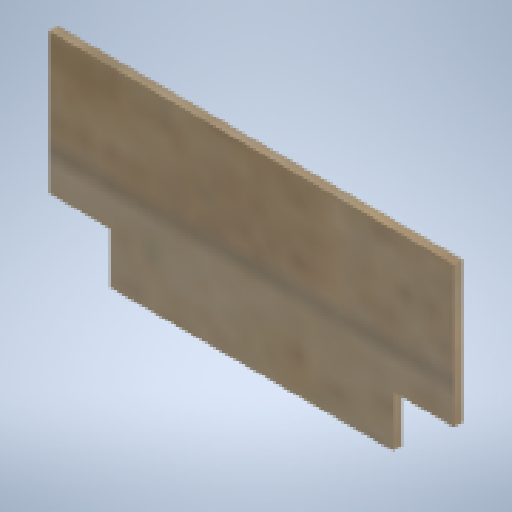
# Autodesk Inventor part: wall
Saved by Autodesk Inventor 2026.1 (Build 301233020, 233B)
## iProperties
Created: 2025-11-03
Part Number: wall
Material: 木材 (カエデ材)
Document SubType Name: Modeling
Designer: hibik
Density: 0.67 g/cm^3
Appearance: ナチュラル カエデ材 - 光沢 濃い着色
Author: hibik
Autodesk Inventor part; units mm, degrees
ref_plane "YZ Plane" through (0, 0, 0) normal (1, 0, 0) x (0, 1, 0)
ref_plane "XZ Plane" through (0, 0, 0) normal (0, 1, 0) x (-1, 0, 0)
ref_plane "XY Plane" through (0, 0, 0) normal (0, 0, 1) x (1, 0, 0)
sketch "スケッチ1" plane through (0, 0, 0) normal (0, 0, 1) x (1, 0, 0)
  line L0 (-40.22, 0) -> (40.22, 0)
  line L1 (40.22, 0) -> (40.22, 14.5)
  line L2 (40.22, 14.5) -> (-40.22, 14.5)
  line L3 (-40.22, 14.5) -> (-40.22, 0)
  line L4 (-57.5, 14.5) -> (57.5, 14.5)
  line L5 (57.5, 14.5) -> (57.5, 54.5)
  line L6 (57.5, 54.5) -> (-57.5, 54.5)
  line L7 (-57.5, 54.5) -> (-57.5, 14.5)
  point P0 (0, 0)
  point P1 (0, 0)
  point P2 (0, 14.5)
  dimension "d0" = 80.44
  dimension "d1" = 14.5
  dimension "d2" = 115
  dimension "d3" = 40
  constraints: 16 end point, 4 parallel, 3 midpoint, 2 horizontal, 2 perpendicular, 1 coincident
  measures "d0" distance of L0.start L0.end
  measures "d1" distance of L2.end L0.start
  measures "d2" distance of L5.end L6.end
  measures "d3" distance of L6.end L4.start
extrude "押し出し1" add sketch "スケッチ1" along normal blind 2.5
